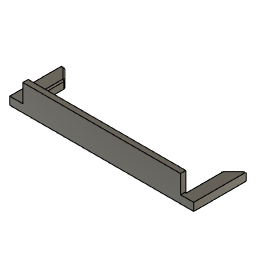
Bot_Dispensor_holder (Autodesk Fusion 360 design; units mm, degrees)
Autodesk Fusion 360 part; units mm, degrees
sketch "Sketch1" plane through (0, 0, 0) normal (0, 0, 1) x (1, 0, 0)
  line L0 (0, 0) -> (70, 0)
  line L1 (70, 0) -> (70, 20)
  line L2 (70, 20) -> (0, 20)
  line L3 (0, 20) -> (0, 0)
  line L4 (35, 0) -> (35, 2)
  line L5 (35, 2) -> (5, 2)
  line L6 (5, 2) -> (5, 20)
  line L7 (65, 2) -> (65, 20)
  line L8 (35, 2) -> (65, 2)
  line L9 (5, 2) -> (5, 0)
  line L10 (65, 2) -> (65, 0)
  dimension "d2" = 70
  dimension "d3" = 20
  dimension "d5" = 2
  dimension "d6" = 30
  constraint horizontal L0
  constraint vertical L1
  constraint horizontal L2
  constraint vertical L3
  constraint coincident L0.start L3.end
  constraint midpoint L0 L4.start
  constraint perpendicular L0 L4
  constraint perpendicular L4 L5
  constraint coincident L2 L6.end
  constraint perpendicular L2 L6
  constraint symmetric L5.start L4 L8.start
  constraint symmetric L4 L5.end L7.start
  constraint symmetric L4 L6.end L7.end
  constraint coincident L0 L9.end
  constraint perpendicular L0 L9
  constraint coincident L0 L10.end
  constraint perpendicular L0 L10
  measures "d2" distance of L0.start L0.end
  measures "d3" distance of L0.start L2.end
  measures "d5" distance of L4.start L4.end
  measures "d6" distance of L4.end L5.end
extrude "Extrude1" add sketch "Sketch1" along normal blind 3 contours L0 L2 L3 L6 L9 | L0 L4 L5 L9 | L0 L4 L8 L10 | L0 L1 L2 L7 L10
chamfer "Chamfer1" distance 4 distance2 4 1 edges at (65, 20, 1.5) measured on face at (68.3333, 20, 1)
chamfer "Chamfer1" distance 4 distance2 4 1 edges at (5, 20, 1.5) measured on face at (5, 8, 1)
fillet "Fillet1" radius 1 4 edges at (5, 16, 1.5) (1, 20, 1.5) (65, 16, 1.5) (69, 20, 1.5)
fillet "Fillet2" radius 0.5 9 edges at (35, 2, 3) (69.0315, 19.9239, 3) (67, 18, 3) (65.0761, 15.9685, 3) (65, 8.7929, 3) (5, 8.7929, 3) (4.9239, 15.9685, 3) (3, 18, 3) (0.9685, 19.9239, 3)
extrude "Extrude2" add sketch "Sketch1" along normal blind 10 contours L0 L4 L5 L9 | L0 L4 L8 L10
equation "box_width = 70 mm"
equation "d2 = box_width"
equation "d3 = box_len"
equation "cover_width = 60 mm"
equation "d6 = cover_width / 2"
equation "box_len = 20 mm"
